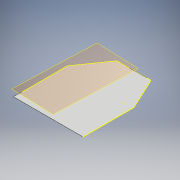
# Autodesk Inventor part: cover end plates-01
Saved by Autodesk Inventor 2018 (Build 220112000, 112)
## iProperties
Created: 2018-05-29
Part Number: cover end plates-01
Material: Generic
Document SubType Name: Modeling
Designer: P446509
Density: 1 g/cm^3
Appearance: Default
Author: P446509
Autodesk Inventor part; units mm, degrees
ref_plane "YZ Plane" through (0, 0, 0) normal (1, 0, 0) x (0, 1, 0)
ref_plane "XZ Plane" through (0, 0, 0) normal (0, 1, 0) x (-1, 0, 0)
ref_plane "XY Plane" through (0, 0, 0) normal (0, 0, 1) x (1, 0, 0)
ref_plane "Work Plane1" through (-527.421, 38.0398, -128.7467) normal (0, 0, 1) x (0.9993843, -0.0350873, 0)
sketch "Sketch1" plane through (-527.421, 38.0398, -128.7467) normal (0, 0, 1) x (0.9993843, -0.0350873, 0)
  line L0 (-71.9298, -7.1441) -> (116.8182, 283.622) projected
  line L1 (116.8182, 283.622) -> (240.6596, 287.9699) projected
  line L2 (449.4274, 297.701) -> (252.1683, 290.7755) projected
  line L3 (607.7587, -12.8972) -> (449.4274, 297.701) projected
  line L4 (625.2338, -510.6359) -> (607.7587, -12.8972) projected
  line L5 (-56.2402, -454.0286) -> (-71.9298, -7.1441) projected
  point P0 (528.431, -19.5106)
sketch "Sketch2" plane through (-527.421, 38.0398, -128.7467) normal (0, 0, 1) x (0.9993843, -0.0350873, 0)
  line L0 (-71.9298, -7.1441) -> (116.8182, 283.622) projected
  line L1 (-56.2402, -454.0286) -> (-71.9298, -7.1441) projected
  line L2 (116.8182, 283.622) -> (240.6596, 287.9699) projected
  line L3 (607.7587, -12.8972) -> (449.4274, 297.701) projected
  line L4 (625.2338, -510.6359) -> (607.7587, -12.8972) projected
  line L5 (625.2338, -510.6359) -> (-56.2402, -534.5617)
  line L6 (-56.2402, -534.5617) -> (-56.2402, -454.0286)
  line L7 (116.8182, 283.622) -> (449.4274, 297.701)
  point P0 (528.431, -19.5106)
  constraints: 6 end point, 1 vertical
extrude "Extrusion1" add sketch "Sketch2" against normal blind 1.6
body "Solid1"
